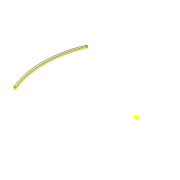
# Autodesk Inventor part: Part_13
Saved by Autodesk Inventor 2022 (Build 260153000, 153)
## iProperties
Created: 2022-04-26
Part Number: Part_13
Material: Generic
Document SubType Name: Modeling
Designer: dell
Density: 1 g/cm^3
Appearance: Default
Author: dell
Autodesk Inventor part; units mm, degrees
ref_plane "YZ Plane" through (0, 0, 0) normal (1, 0, 0) x (0, 1, 0)
ref_plane "XZ Plane" through (0, 0, 0) normal (0, 1, 0) x (-1, 0, 0)
ref_plane "XY Plane" through (0, 0, 0) normal (0, 0, 1) x (1, 0, 0)
sketch "Sketch1" plane through (0, 0, 0) normal (0, 1, 0) x (-1, 0, 0)
  line L0 (0, 0) -> (0, -382.775) construction
  line L1 (-5, 0) -> (-5, -382.775)
  line L2 (5, -382.775) -> (5, 0)
  arc A0 (5, 0) -> (-5, 0) centre (0, 0) ccw
  arc A1 (-5, -382.775) -> (5, -382.775) centre (0, -382.775) ccw
  circle A2 centre (0, 0) radius 1.5
  circle A3 centre (0, -382.775) radius 1.5
  arc A4 (5, -382.775) -> (5, 0) centre (-456.9208, -191.3875) ccw
  arc A5 (-5, -382.775) -> (-5, 0) centre (-466.9208, -191.3875) ccw
  point P0 (0, -191.3875)
  dimension "d0" = 382.775
  dimension "d1" = 10
  dimension "d2" = 3
  dimension "d3" = 3
  dimension "d12" = 500
  dimension "d13" = 500
  constraints: 8 end point, 8 point on circle, 6 centre point, 4 tangent, 2 coincident, 1 midpoint, 1 parallel, 1 vertical
  measures "d0" distance of L0.start L0.end
  measures "d1" diameter of A1
  measures "d2" diameter of A2
  measures "d3" diameter of A3
  measures "d12" radius of A4
  measures "d13" radius of A5
extrude "Extrusion1" add sketch "Sketch1" along normal blind 8 contours A0 L2 A5 | A5 L2 A1 | A4 L2 A5
sketch "Sketch2" plane through (0, 0, 0) normal (0, -1, 0) x (1, 0, 0)
  arc A0 (-5, -382.775) -> (5, -382.775) centre (0, -382.775) ccw projected
  arc A1 (5, 0) -> (-5, 0) centre (0, 0) ccw projected
  circle A2 centre (0, -382.775) radius 1.5 projected
  circle A3 centre (0, 0) radius 1.5 projected
  arc A4 (-5, 0) -> (-5, -382.775) centre (456.9208, -191.3875) ccw projected
  arc A5 (5, 0) -> (5, -382.775) centre (466.9208, -191.3875) ccw projected
fillet "Fillet1" radius 2 4 edges at (5, 4, -382.775) (-5, 4, -382.775) (-5, 4, 0) (5, 4, 0)
body "Solid1"
